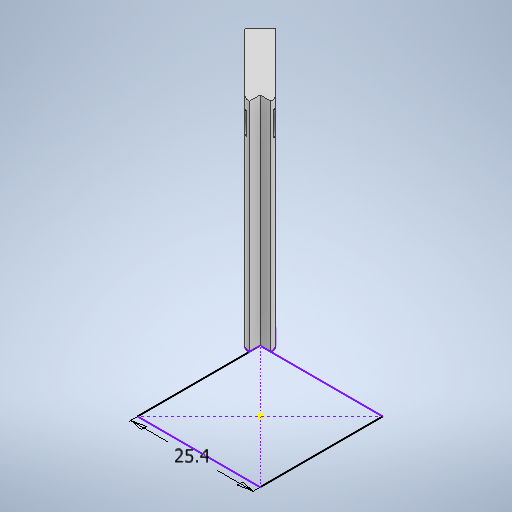
# Autodesk Inventor part: Gripper_Gen3_FingerRail
Saved by Autodesk Inventor 2025.1 (Build 291241000, 241)
## iProperties
Created: 2024-10-29
Part Number: Gripper_Gen3_FingerRail
Material: Generic
Document SubType Name: Modeling
Designer: m_kni
Density: 1 g/cm^3
Appearance: Default
Author: m_kni
Autodesk Inventor part; units mm, degrees
ref_plane "YZ Plane" through (0, 0, 0) normal (1, 0, 0) x (0, 1, 0)
ref_plane "XZ Plane" through (0, 0, 0) normal (0, 1, 0) x (-1, 0, 0)
ref_plane "XY Plane" through (0, 0, 0) normal (0, 0, 1) x (1, 0, 0)
sketch "Sketch1" plane through (0, 0, 0) normal (0, 1, 0) x (-1, 0, 0)
  line L0 (-12.7, -12.7) -> (10.45, -12.7)
  line L1 (12.7, -10.45) -> (12.7, 12.7)
  line L2 (12.7, 12.7) -> (-12.7, 12.7)
  line L3 (-12.7, 12.7) -> (-12.7, -12.7)
  line L4 (-12.7, -12.7) -> (12.7, 12.7) construction
  line L5 (12.7, -12.7) -> (-12.7, 12.7) construction
  line L6 (17.473, -17.473) -> (23.3066, -23.3066)
  arc A0 (14.291, -17.473) -> (17.473, -14.291) centre (15.882, -15.882) ccw
  line L7 (14.291, -11.109) -> (17.473, -14.291)
  line L8 (11.109, -14.291) -> (14.291, -17.473)
  line L9 (12.7, -10.45) -> (12.7, -12.7)
  line L10 (12.7, -12.7) -> (10.45, -12.7)
  arc A1 (14.291, -11.109) -> (12.7, -10.45) centre (12.7, -12.7) ccw
  arc A2 (10.45, -12.7) -> (11.109, -14.291) centre (12.7, -12.7) ccw
  point P0 (0, 0)
  point P1 (15.882, -15.882)
  dimension "d0" = 25.4
  constraints: 22 end point, 8 point on circle, 3 centre point, 3 parallel, 2 midpoint, 1 coincident, 1 horizontal, 1 perpendicular, 1 point on line
  measures "d0" distance of L2.end L1.end
extrude "Extrusion1" add sketch "Sketch1" along normal blind 45 contours L10 L9 A1 L7 A0 L8 A2
sketch "Sketch2" plane through (0, 45, 0) normal (0, 1, 0) x (1, 0, 0)
  arc A0 (-14.291, 11.109) -> (-12.7, 10.45) centre (-12.7, 12.7) ccw projected
  line L0 (-12.7, 10.45) -> (-12.7, 12.7) projected
  line L1 (-12.7, 12.7) -> (-10.45, 12.7) projected
  arc A1 (-10.45, 12.7) -> (-11.109, 14.291) centre (-12.7, 12.7) ccw projected
  line L2 (-11.109, 14.291) -> (-14.291, 17.473) projected
  arc A2 (-14.291, 17.473) -> (-17.473, 14.291) centre (-15.882, 15.882) ccw projected
  line L3 (-17.473, 14.291) -> (-14.291, 11.109) projected
  line L4 (-17.473, 17.473) -> (-15.882, 19.064)
  arc A3 (-14.291, 17.473) -> (-17.473, 14.291) centre (-15.882, 15.882) ccw projected
  line L5 (-15.882, 19.064) -> (-19.064, 15.882)
  line L6 (-19.064, 15.882) -> (-14.291, 11.109)
  line L7 (-14.291, 11.109) -> (-11.109, 14.291)
  line L8 (-11.109, 14.291) -> (-15.882, 19.064)
  line L9 (-19.064, 15.882) -> (-26.135, 22.953)
  line L10 (-15.882, 19.064) -> (-22.953, 26.135)
  line L11 (-22.953, 26.135) -> (-26.135, 22.953)
  point P0 (0, 0)
  dimension "d10" = 10
  constraints: 16 end point, 3 perpendicular, 3 point on line, 1 collinear, 1 point on circle, 1 tangent
  measures "d10" distance of L5.end L9.end
extrude "Extrusion2" add sketch "Sketch2" against normal blind 9 contours L3 A2 L2 L7 | L6 L5 A2 | L4 L8 A2 | L5 L9 L11 L10 L4
sketch "Sketch3" plane through (-22.953, 36, -26.135) normal (-0.7071, 0, -0.7071) x (-0.7071, 0, 0.7071)
  line L0 (0, 0) -> (4.5, 0) projected
  line L1 (4.5, 9) -> (4.5, 0)
  line L2 (4.5, -36) -> (4.5, 9) projected
  line L3 (0, 9) -> (4.5, 9) projected
  line L4 (4.25, 2.2514) -> (4.75, 2.2514)
  line L5 (4.75, 2.2514) -> (4.75, 6.7486)
  line L6 (4.75, 6.7486) -> (4.25, 6.7486)
  line L7 (4.25, 6.7486) -> (4.25, 2.2514)
  line L8 (4.25, 2.2514) -> (4.75, 6.7486) construction
  line L9 (4.75, 2.2514) -> (4.25, 6.7486) construction
  line L10 (-0.25, 2) -> (0.25, 2)
  line L11 (0.25, 2) -> (0.25, 7)
  line L12 (0.25, 7) -> (-0.25, 7)
  line L13 (-0.25, 7) -> (-0.25, 2)
  line L14 (0, -36) -> (0, 9) projected
  line L15 (-0.25, 2) -> (0.25, 7) construction
  line L16 (0.25, 2) -> (-0.25, 7) construction
  line L17 (4.5, 6.7486) -> (4.5, 2.2514)
  line L18 (0, 2) -> (0, 7)
  point P0 (2.25, -36)
  point P1 (4.5, 4.5)
  point P2 (0, 4.5)
  dimension "d13" = 9
  dimension "d14" = 4.5
  dimension "d15" = 4.5
  dimension "d16" = 0.5
  dimension "d17" = 0.5
  dimension "d18" = 5
  constraints: 30 end point, 8 midpoint, 4 parallel, 4 point on line, 2 horizontal, 2 perpendicular, 1 vertical
  measures "d13" distance of L0.end L1.start
  measures "d14" distance of point (4.5, 4.5) L0.end
  measures "d15" distance of L3.start L1.start
  measures "d16" distance of L6.end L5.end
  measures "d17" distance of L12.end L11.end
  measures "d18" distance of L11.end L10.end
extrude "Extrusion3" cut sketch "Sketch3" against normal blind 21.7 contours L14 L12 L11 L10 | L10 L13 L12 L14 | L4 L7 L6 L1 | L1 L6 L5 L4
body "Solid1"
